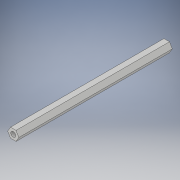
# Autodesk Inventor part: trudong
Saved by Autodesk Inventor 2019 (Build 230136000, 136)
## iProperties
Created: 2021-01-20
Part Number: trudong
Material: Generic
Document SubType Name: Modeling
Designer: Admin
Density: 1 g/cm^3
Appearance: Default
Author: Admin
Autodesk Inventor part; units mm, degrees
ref_plane "YZ Plane" through (0, 0, 0) normal (1, 0, 0) x (0, 1, 0)
ref_plane "XZ Plane" through (0, 0, 0) normal (0, 1, 0) x (-1, 0, 0)
ref_plane "XY Plane" through (0, 0, 0) normal (0, 0, 1) x (1, 0, 0)
sketch "Sketch1" plane through (0, 0, 0) normal (0, 0, 1) x (1, 0, 0)
  circle A0 centre (0, 0) radius 1.5
  line L0 (3.431, 0) -> (1.7155, -2.9714)
  line L1 (1.7155, -2.9714) -> (-1.7155, -2.9714)
  line L2 (-1.7155, -2.9714) -> (-3.431, 0)
  line L3 (-3.431, 0) -> (-1.7155, 2.9714)
  line L4 (-1.7155, 2.9714) -> (1.7155, 2.9714)
  line L5 (1.7155, 2.9714) -> (3.431, 0)
  dimension "d0" = 3
  constraints: 12 end point, 2 coincident, 1 centre point, 13 other
  measures "d0" diameter of A0
extrude "Extrusion1" add sketch "Sketch1" along normal blind 95
body "Solid1"
